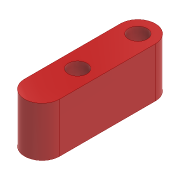
# Autodesk Inventor part: Limit switch trigger spacer extension arm
Saved by Autodesk Inventor 2020 (Build 240168000, 168)
## iProperties
Created: 2019-11-21
Part Number: Limit switch trigger spacer extension arm
Material: Generic
Document SubType Name: Modeling
Designer: ball
Density: 1 g/cm^3
Appearance: Default
Author: ball
Autodesk Inventor part; units mm, degrees
ref_plane "YZ Plane" through (0, 0, 0) normal (1, 0, 0) x (0, 1, 0)
ref_plane "XZ Plane" through (0, 0, 0) normal (0, 1, 0) x (-1, 0, 0)
ref_plane "XY Plane" through (0, 0, 0) normal (0, 0, 1) x (1, 0, 0)
sketch "Sketch1" plane through (0, 0, 0) normal (0, 1, 0) x (-1, 0, 0)
  circle A0 centre (0, 0) radius 1.7
  arc A1 (-3.175, 0) -> (3.175, 0) centre (0, 0) ccw
  line L0 (-3.175, 0) -> (-3.175, 17.399)
  line L1 (3.175, 17.399) -> (3.175, 0)
  arc A2 (3.175, 17.399) -> (-3.175, 17.399) centre (0, 17.399) ccw
  circle A3 centre (0, 10.9474) radius 1.7
  dimension "d0" = 3.4
  dimension "d1" = 6.35
  dimension "d6" = 6.35
  dimension "d8" = 17.399
  dimension "d9" = 3.4
  dimension "d10" = 10.9474
  constraints: 4 centre point, 4 end point, 4 point on circle, 2 coincident, 1 parallel
  measures "d0" diameter of A0
  measures "d1" diameter of A1
  measures "d6" diameter of A2
  measures "d8" distance of A2.centre point (0, 0)
  measures "d9" diameter of A3
  measures "d10" distance of A3.centre point (0, 0)
extrude "Extrusion1" add sketch "Sketch1" along normal blind 9
body "Solid1"
